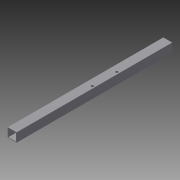
# Autodesk Inventor part: Square Motor Mount
Saved by Autodesk Inventor 2013 (Build 170138000, 138)
## iProperties
Created: 2013-01-21
Part Number: Square Motor Mount
Material: Aluminum 6061
Document SubType Name: Modeling
Designer: actoennies
Density: 2.71 g/cm^3
Mass: 181.529 g
Surface Area: 848.276 cm^2
Volume: 66.9849 cm^3
Author: actoennies
Autodesk Inventor part; units mm, degrees
ref_plane "YZ Plane" through (0, 0, 0) normal (1, 0, 0) x (0, 1, 0)
ref_plane "XZ Plane" through (0, 0, 0) normal (0, 1, 0) x (-1, 0, 0)
ref_plane "XY Plane" through (0, 0, 0) normal (0, 0, 1) x (1, 0, 0)
sketch "Sketch1" plane through (0, 0, 0) normal (0, 0, 1) x (1, 0, 0)
  line L0 (0, 0) -> (-25.4, 0)
  line L1 (-25.4, 0) -> (-25.4, 25.4)
  line L2 (-25.4, 25.4) -> (0, 25.4)
  line L3 (0, 25.4) -> (0, 0)
  line L4 (-1.5875, 23.8125) -> (-23.8125, 23.8125)
  line L5 (-23.8125, 23.8125) -> (-23.8125, 1.5875)
  line L6 (-23.8125, 1.5875) -> (-1.5875, 1.5875)
  line L7 (-1.5875, 1.5875) -> (-1.5875, 23.8125)
  dimension "d0" = 25.4
  dimension "d2" = 25.4
  dimension "d3" = 1.5875
  constraints: 16 end point, 4 parallel, 2 perpendicular, 1 horizontal, 3 other
  measures "d0" distance of L1.end L2.end
  measures "d2" distance of L2.end L0.start
  measures "d3" distance between parallel lines of L2 L4
extrude "Extrusion1" add sketch "Sketch1" along normal blind 508
sketch "Sketch2" plane through (-25.4, 25.4, 0) normal (0, 1, 0) x (1, 0, 0)
  line L0 (0, 0) -> (25.4, 0) projected
  line L1 (0, 0) -> (0, -508) projected
  line L2 (25.4, -508) -> (0, -508) projected
  line L3 (25.4, 0) -> (25.4, -508) projected
  line L4 (0, -63.5) -> (25.4, -63.5) construction
  line L5 (0, -63.5) -> (25.4, -63.5)
  point P0 (25.4, -54.61)
  point P1 (0, -56.388)
  point P2 (25.4, -60.1453)
  dimension "d12" = 3.3547
  dimension "d13" = 444.5
  constraints: 5 point on line, 4 end point, 1 collinear, 1 perpendicular
  measures "d12" distance of L4.end point (25.4, -60.145)
  measures "d13" distance from line of L2 L4.start
extrude "Extrusion2" cut sketch "Sketch2" against normal blind 508 contours L0 L3 L5 L1
sketch "Sketch3" plane through (-25.4, 0, 508) normal (0, -1, 0) x (1, 0, 0)
  circle A0 centre (12.7, -235.8157) radius 3.3782
  circle A1 centre (12.7, -305.6657) radius 3.3782
  point P0 (25.4, -508)
  constraints: 2 centre point, 4 other
extrude "Extrusion3" cut sketch "Sketch3" against normal blind 25.4
body "Solid1"
